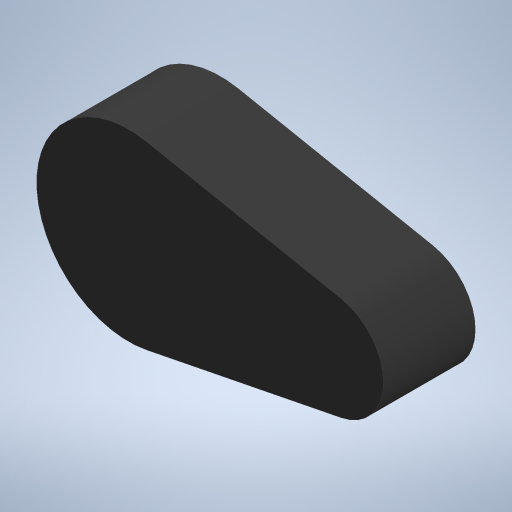
# Autodesk Inventor part: Joystick base
Saved by Autodesk Inventor 2023 (Build 270158000, 158)
## iProperties
Created: 2023-11-16
Part Number: Joystick base
Material: ABS Plastic
Document SubType Name: Modeling
Designer: DELL
Density: 1.06 g/cm^3
Appearance: Smooth - White
Author: DELL
Autodesk Inventor part; units mm, degrees
ref_plane "YZ Plane" through (0, 0, 0) normal (1, 0, 0) x (0, 1, 0)
ref_plane "XZ Plane" through (0, 0, 0) normal (0, 1, 0) x (-1, 0, 0)
ref_plane "XY Plane" through (0, 0, 0) normal (0, 0, 1) x (1, 0, 0)
sketch "Sketch1" plane through (0, 0, 0) normal (0, 0, 1) x (1, 0, 0)
  arc A0 (6.8099, 34.3311) -> (6.8099, -34.3311) centre (0, 0) ccw
  circle A1 centre (115.45, 0) radius 0.0883
  arc A2 (80.9848, -19.6178) -> (80.9848, 19.6178) centre (77.0934, 0) ccw
  line L0 (6.8099, 34.3311) -> (80.9848, 19.6178)
  line L1 (115.3617, 0) -> (115.5383, 0)
  line L2 (6.8099, -34.3311) -> (80.9848, -19.6178)
  point P0 (-20.5004, 39.7484)
  point P1 (110.1386, 13.8348)
  point P2 (-20.5004, -39.7484)
  point P3 (110.1386, -13.8348)
  point P4 (97.0934, 0)
  point P5 (-35, 0)
  dimension "d0" = 70
  dimension "d2" = 40
  dimension "d3" = 0
  dimension "d4" = 132.0934
  constraints: 8 point on circle, 6 end point, 3 centre point, 2 symmetric about line, 2 tangent, 1 coincident, 1 horizontal
  measures "d0" diameter of A0
  measures "d2" diameter of A2
  measures "d3" vertical distance of point (0, 0) A2.centre
  measures "d4" distance of point (97.093, 0) point (-35, 0)
extrude "Extrusion1" add sketch "Sketch1" along normal blind 35 contours L0 A2 L2 A0
body "Solid1"
